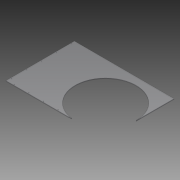
# Autodesk Inventor part: Hopper Bottom
Saved by Autodesk Inventor 2014 SP1 (Build 180222100, 222)
## iProperties
Created: 2013-12-16
Part Number: Hopper Bottom
Material: Polycarbonate, Clear
Document SubType Name: Modeling
Designer: Moses
Mass: 320.283 g
Surface Area: 1746.68 cm^2
Volume: 266.903 cm^3
Density: 1.2 g/cm^3
Appearance: Polycarbonate - Clear
Author: Moses
Autodesk Inventor part; units mm, degrees
ref_plane "YZ Plane" through (0, 0, 0) normal (1, 0, 0) x (0, 1, 0)
ref_plane "XZ Plane" through (0, 0, 0) normal (0, 1, 0) x (-1, 0, 0)
sketch "Sketch1" plane through (0, 0, 0) normal (0, 1, 0) x (-1, 0, 0)
  arc A0 (0, 180.975) -> (146.05, 327.025) centre (146.05, 180.975) ccw
  line L0 (0, 180.975) -> (0, 0)
  line L1 (0, 0) -> (476.25, 0)
  line L2 (476.25, 0) -> (476.25, 327.025)
  line L3 (476.25, 327.025) -> (146.05, 327.025)
  circle A1 centre (301.625, 322.6594) radius 1.5875 projected
  circle A2 centre (441.325, 322.6594) radius 1.5875 projected
  circle A3 centre (371.475, 322.6594) radius 1.5875 projected
  circle A4 centre (231.775, 322.6594) radius 1.5875 projected
  line L4 (450.85, 330.2) -> (450.85, 315.1187) construction
  line L5 (450.85, 330.2) -> (222.25, 330.2) construction
  line L6 (222.25, 315.1187) -> (222.25, 330.2) construction
  line L7 (450.85, 315.1187) -> (222.25, 315.1187) construction
  line L8 (152.5101, 326.2312) -> (152.5101, 327.025) construction
  line L9 (152.5101, 326.2312) -> (177.4637, 326.2312) construction
  line L10 (177.4637, 327.025) -> (177.4637, 326.2312) construction
  line L11 (152.5101, 327.025) -> (177.4637, 327.025) construction
  line L12 (177.4637, 327.025) -> (177.4637, 326.009)
  line L13 (177.4637, 326.009) -> (163.2471, 326.009)
  arc A5 (163.2471, 326.009) -> (146.05, 327.025) centre (146.05, 180.975) ccw
  line L14 (146.05, 327.025) -> (177.4637, 327.025)
  dimension "d0" = 327.025
  dimension "d1" = 330.2
  dimension "d2" = 476.25
  dimension "d3" = 146.05
  dimension "d4" = 180.975
  dimension "d9" = 1.016
  constraints: 14 end point, 5 point on circle, 2 centre point, 2 horizontal, 2 perpendicular, 2 vertical, 1 coincident, 1 concentric
  measures "d0" distance of L1.end L2.end
  measures "d1" distance of L2.end L3.end
  measures "d2" distance of L0.end L1.end
  measures "d3" radius of A0
  measures "d4" distance of L0.start L0.end
  measures "d9" distance of L10.start L12.end
extrude "Extrusion1" add sketch "Sketch1" along normal blind 3.175 contours A0 L13 L12 L3 L2 L1 L0
ref_plane "Work Plane1" through (-464.1307, 0, 8.7312) normal (-0.1867, 0.9824, 0) x (-0.9824, -0.1867, 0)
sketch "Sketch2" plane through (-464.1307, 0, 8.7312) normal (-0.1867, 0.9824, 0) x (-0.9824, -0.1867, 0)
  circle A0 centre (7.5406, 223.8375) radius 1.5875 projected
  circle A1 centre (7.5406, 80.9625) radius 1.5875 projected
  circle A2 centre (7.5406, 9.525) radius 1.5875 projected
  circle A3 centre (7.5406, 152.4) radius 1.5875 projected
  circle A4 centre (7.5406, 295.275) radius 1.5875 projected
  line L0 (15.0813, 0) -> (0, 0) construction
  line L1 (15.0813, 0) -> (15.0813, 304.8) construction
  line L2 (0, 304.8) -> (15.0813, 304.8) construction
  line L3 (0, 0) -> (0, 304.8) construction
  point P0 (-455.9729, -8.7312)
extrude "Extrusion2" cut sketch "Sketch2" along normal through all
body "Solid1"
